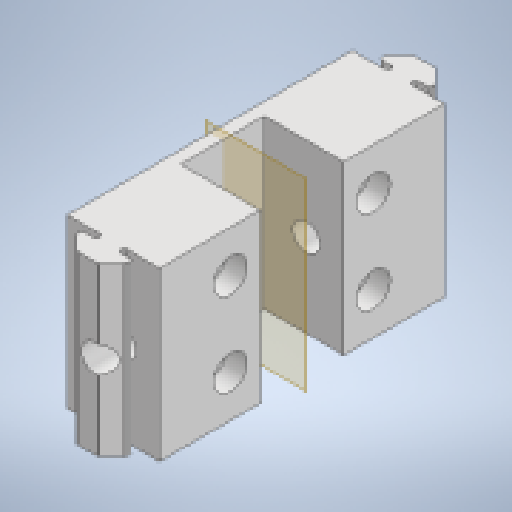
# Autodesk Inventor part: linac_upper_holder
Saved by Autodesk Inventor 2024 (Build 280153000, 153)
## iProperties
Created: 2025-12-26
Part Number: linac_upper_holder
Material: Generic
Document SubType Name: Modeling
Designer: schar
Density: 1 g/cm^3
Appearance: Default
Author: schar
Autodesk Inventor part; units mm, degrees
ref_plane "YZ Plane" through (0, 0, 0) normal (1, 0, 0) x (0, 1, 0)
ref_plane "XZ Plane" through (0, 0, 0) normal (0, 1, 0) x (-1, 0, 0)
sketch "Sketch1" plane through (0, 0, 0) normal (1, 0, 0) x (0, 1, 0)
  line L0 (20, 27.056) -> (-20, 27.056)
  line L1 (-20, 27.056) -> (-20, -27.056)
  line L2 (-20, -27.056) -> (20, -27.056)
  line L3 (20, -27.056) -> (20, 27.056)
  line L4 (20, 27.056) -> (-20, -27.056) construction
  line L5 (-20, 27.056) -> (20, -27.056) construction
  point P0 (0, 0)
  dimension "d0" = 40
  dimension "d1" = 54.112
  constraints: 12 end point, 2 midpoint, 2 parallel, 1 horizontal, 1 perpendicular
  measures "d0" distance of L2.end L1.end
  measures "d1" distance of L1.end L0.end
extrude "Extrusion1" add sketch "Sketch1" along normal blind 4
sketch "Sketch2" plane through (4, 0, 0) normal (1, 0, 0) x (0, 0, -1)
  line L0 (-9, 9) -> (9, 9)
  line L1 (9, 9) -> (9, -9)
  line L2 (9, -9) -> (-9, -9)
  line L3 (-9, -9) -> (-9, 9)
  line L4 (-9, 9) -> (9, -9) construction
  line L5 (9, 9) -> (-9, -9) construction
  line L6 (-27.056, -20) -> (27.056, -20) projected
  line L7 (-27.056, 20) -> (27.056, 20)
  line L8 (27.056, 20) -> (27.056, -20)
  line L9 (27.056, -20) -> (-27.056, -20)
  line L10 (-27.056, -20) -> (-27.056, 20)
  line L11 (-27.056, 20) -> (27.056, -20) construction
  line L12 (27.056, 20) -> (-27.056, -20) construction
  point P0 (0, 0)
  dimension "d4" = 18
  dimension "d5" = 18
  constraints: 24 end point, 4 midpoint, 4 parallel, 2 horizontal, 2 perpendicular
  measures "d4" distance of L1.end L2.end
  measures "d5" distance of L0.end L1.end
extrude "Extrusion2" add sketch "Sketch2" along normal blind 18
sketch "Sketch3" plane through (22, 0, 0) normal (1, 0, 0) x (0, 0, -1)
  line L0 (9, -9) -> (-9, -9) projected
  line L1 (-27.056, -20) -> (27.056, -20) projected
  line L2 (-9, -9) -> (9, -9)
  line L3 (9, -9) -> (9, -20)
  line L4 (9, -20) -> (-9, -20)
  line L5 (-9, -20) -> (-9, -9)
  point P0 (0, 0)
  dimension "d8" = 18
  constraints: 8 end point, 2 parallel, 1 horizontal, 1 perpendicular, 1 point on line
  measures "d8" distance of L3.end L4.end
extrude "Extrusion3" cut sketch "Sketch3" against normal blind 18
sketch "Sketch4" plane through (22, 0, 0) normal (1, 0, 0) x (0, 0, -1)
  line L0 (-27.056, 20) -> (-27.056, -20) projected
  line L1 (-27.056, -20) -> (-17.056, -20)
  line L2 (-27.056, -20) -> (27.056, -20) projected
  line L3 (-17.056, -20) -> (-17.056, -10)
  line L4 (-27.056, 20) -> (-17.056, 20)
  line L5 (27.056, 20) -> (-27.056, 20) projected
  line L6 (-17.056, 20) -> (-17.056, 10)
  line L7 (27.056, -20) -> (27.056, 20) projected
  line L8 (27.056, 20) -> (27.056, 10)
  line L9 (27.056, 10) -> (17.056, 10)
  line L10 (27.056, -20) -> (27.056, -10)
  line L11 (27.056, -10) -> (17.056, -10)
  circle A0 centre (-17.056, 10) radius 2.5
  circle A1 centre (-17.056, -10) radius 2.5
  circle A2 centre (17.056, 10) radius 2.5
  circle A3 centre (17.056, -10) radius 2.5
  point P0 (0, 0)
  dimension "d11" = 10
  dimension "d12" = 10
  dimension "d13" = 10
  dimension "d14" = 10
  dimension "d15" = 10
  dimension "d16" = 10
  dimension "d17" = 10
  dimension "d18" = 10
  dimension "d19" = 5
  dimension "d20" = 5
  dimension "d21" = 5
  dimension "d22" = 5
  constraints: 16 end point, 4 centre point, 4 coincident, 4 point on line, 3 perpendicular, 1 vertical
  measures "d11" distance of L0.end L1.end
  measures "d12" distance of L1.end L3.end
  measures "d13" distance of L0.start L4.end
  measures "d14" distance of L4.end L6.end
  measures "d15" distance of L5.start L8.end
  measures "d16" distance of L8.end L9.end
  measures "d17" distance of L2.end L10.end
  measures "d18" distance of L10.end L11.end
  measures "d19" diameter of A0
  measures "d20" diameter of A1
  measures "d21" diameter of A2
  measures "d22" diameter of A3
extrude "Extrusion4" cut sketch "Sketch4" against normal through all contours A0 | A1 | A2 | A3
sketch "Sketch6" plane through (0, -20, -27.056) normal (0, 0, -1) x (-1, 0, 0)
  line L0 (0, 20) -> (-22, 20)
  line L1 (-22, 20) -> (-13, 20)
  circle A0 centre (-13, 20) radius 3.25
  dimension "d32" = 22
  dimension "d33" = 9
  dimension "d34" = 6.5
  constraints: 4 end point, 1 centre point, 1 coincident, 1 horizontal, 1 point on line
  measures "d32" distance of L0.start L0.end
  measures "d33" distance of L0.end L1.end
  measures "d34" diameter of A0
extrude "Extrusion5" cut sketch "Sketch6" against normal through all
sketch "Sketch7" plane through (4, -20, 9) normal (0, 0, -1) x (-1, 0, 0)
  line L0 (0, 29) -> (-18, 29) projected
  line L1 (0, 0) -> (-18, 0)
  line L2 (-18, 0) -> (-18, 29)
  line L3 (-18, 29) -> (0, 29)
  line L4 (0, 29) -> (0, 0)
  point P0 (4, 20)
  constraints: 8 end point, 2 parallel, 1 horizontal, 1 perpendicular
extrude "Extrusion6" cut sketch "Sketch7" against normal blind 1
sketch "Sketch8" plane through (4, -20, -9) normal (0, 0, 1) x (1, 0, 0)
  line L0 (18, 29) -> (18, 0) projected
  line L1 (0, 29) -> (18, 29) projected
  line L2 (18, 0) -> (0, 0)
  line L3 (0, 0) -> (0, 29)
  line L4 (0, 29) -> (18, 29)
  line L5 (18, 29) -> (18, 0)
  point P0 (-4, 20)
  constraints: 8 end point, 2 parallel, 1 horizontal, 1 perpendicular
extrude "Extrusion7" cut sketch "Sketch8" against normal blind 1
sketch "Sketch9" plane through (4, 0, 0) normal (1, 0, 0) x (0, 0, -1)
  line L0 (-10, 9) -> (-10, -20) projected
  line L1 (10, -20) -> (10, 9) projected
  line L2 (-10, 9) -> (10, 9)
  line L3 (10, 9) -> (10, -20)
  line L4 (10, -20) -> (-10, -20)
  line L5 (-10, -20) -> (-10, 9)
  point P0 (0, 0)
  constraints: 8 end point, 2 parallel, 1 horizontal, 1 perpendicular
extrude "Extrusion8" cut sketch "Sketch9" against normal blind 2
sketch "Sketch10" plane through (22, 0, 0) normal (1, 0, 0) x (0, 0, -1)
  circle A0 centre (-17.056, 10) radius 2.5 projected
  circle A1 centre (-17.056, 10) radius 4
  circle A2 centre (17.056, 10) radius 2.5 projected
  circle A3 centre (17.056, 10) radius 4
  circle A4 centre (17.056, -10) radius 2.5 projected
  circle A5 centre (17.056, -10) radius 4
  circle A6 centre (-17.056, -10) radius 2.5 projected
  circle A7 centre (-17.056, -10) radius 4
  point P0 (0, 0)
  dimension "d43" = 8
  dimension "d44" = 8
  dimension "d45" = 8
  dimension "d46" = 8
  constraints: 4 centre point, 4 coincident
  measures "d43" diameter of A1
  measures "d44" diameter of A3
  measures "d45" diameter of A5
  measures "d46" diameter of A7
extrude "Extrusion9" cut sketch "Sketch10" against normal blind 5 contours A0 | A1 | A3 | A5 | A6 | A7
sketch "Sketch11" plane through (22, 9, -10) normal (0, -1, 0) x (1, 0, 0)
  line L0 (0, 0) -> (-20, 0) projected
  line L1 (0, 20) -> (-20, 20)
  line L2 (-20, 20) -> (-20, 0)
  line L3 (-20, 0) -> (0, 0)
  line L4 (0, 0) -> (0, 20)
  point P0 (-22, 10)
  constraints: 8 end point, 2 parallel, 1 horizontal, 1 perpendicular
extrude "Extrusion10" cut sketch "Sketch11" against normal through all
sketch "Sketch12" plane through (0, -20, -27.056) normal (0, 0, -1) x (-1, 0, 0)
  line L0 (0, 0) -> (0, 40) projected
  line L1 (0, 0) -> (-22, 0) projected
  line L2 (0, 40) -> (-22, 40)
  line L3 (-22, 40) -> (-22, 0)
  line L4 (-22, 0) -> (0, 0)
  line L5 (0, 0) -> (0, 40)
  circle A0 centre (-13, 20) radius 3.25 projected
  circle A1 centre (-13, 20) radius 3.25
  point P0 (0, 20)
  constraints: 8 end point, 2 parallel, 1 centre point, 1 coincident, 1 horizontal, 1 perpendicular
extrude "Extrusion11" add sketch "Sketch12" along normal blind 7
sketch "Sketch13" plane through (0, -20, 27.056) normal (0, 0, 1) x (1, 0, 0)
  circle A0 centre (13, 20) radius 3.25 projected
  circle A1 centre (13, 20) radius 3.25
  line L0 (0, 40) -> (0, 0) projected
  line L1 (0, 40) -> (22, 40) projected
  line L2 (0, 0) -> (22, 0)
  line L3 (22, 0) -> (22, 40)
  line L4 (22, 40) -> (0, 40)
  line L5 (0, 40) -> (0, 0)
  point P0 (0, 20)
  constraints: 8 end point, 2 parallel, 1 centre point, 1 coincident, 1 horizontal, 1 perpendicular
extrude "Extrusion12" add sketch "Sketch13" along normal blind 7
sketch "Sketch14" plane through (2, 20, 10) normal (0, 1, 0) x (1, 0, 0)
  arc A0 (9.804, 52.1209) -> (11.1249, 51.7515) centre (10.5684, 52.308) ccw
  line L0 (11.1249, 51.7515) -> (11.3045, 51.9311)
  arc A1 (11.3045, 51.9311) -> (10.9351, 53.252) centre (10.748, 52.4876) ccw
  arc A2 (10.9351, 53.252) -> (10.9351, 54.86) centre (9, 54.056) ccw
  arc A3 (10.9351, 54.86) -> (11.3045, 56.1809) centre (10.748, 55.6244) ccw
  line L1 (11.3045, 56.1809) -> (11.1249, 56.3605)
  arc A4 (11.1249, 56.3605) -> (9.804, 55.9911) centre (10.5684, 55.804) ccw
  arc A5 (9.804, 55.9911) -> (8.196, 55.9911) centre (9, 54.056) ccw
  arc A6 (8.196, 55.9911) -> (6.8751, 56.3605) centre (7.4316, 55.804) ccw
  line L2 (6.8751, 56.3605) -> (6.6955, 56.1809)
  arc A7 (6.6955, 56.1809) -> (7.0649, 54.86) centre (7.252, 55.6244) ccw
  arc A8 (7.0649, 54.86) -> (7.0649, 53.252) centre (9, 54.056) ccw
  arc A9 (7.0649, 53.252) -> (6.6955, 51.9311) centre (7.252, 52.4876) ccw
  line L3 (6.6955, 51.9311) -> (6.8751, 51.7515)
  arc A10 (6.8751, 51.7515) -> (8.196, 52.1209) centre (7.4316, 52.308) ccw
  arc A11 (8.196, 52.1209) -> (9.804, 52.1209) centre (9, 54.056) ccw
  line L4 (18.008, 56.686) -> (18.492, 56.686)
  arc A12 (17.5, 57.194) -> (18.008, 56.686) centre (18.008, 57.194) ccw
  line L5 (17.5, 59.543) -> (17.5, 57.194)
  arc A13 (17.5, 59.543) -> (16.992, 60.051) centre (16.992, 59.543) ccw
  line L6 (16.2661, 60.051) -> (16.992, 60.051)
  arc A14 (16.2661, 60.051) -> (15.9069, 59.9022) centre (16.2661, 59.543) ccw
  line L7 (12.8038, 56.7991) -> (15.9069, 59.9022)
  arc A15 (12.8038, 56.7991) -> (12.655, 56.4399) centre (13.163, 56.4399) ccw
  line L8 (12.655, 51.6721) -> (12.655, 56.4399)
  arc A16 (12.655, 51.6721) -> (12.8038, 51.3129) centre (13.163, 51.6721) ccw
  line L9 (15.9069, 48.2098) -> (12.8038, 51.3129)
  arc A17 (15.9069, 48.2098) -> (16.2661, 48.061) centre (16.2661, 48.569) ccw
  line L10 (16.992, 48.061) -> (16.2661, 48.061)
  arc A18 (16.992, 48.061) -> (17.5, 48.569) centre (16.992, 48.569) ccw
  line L11 (17.5, 50.918) -> (17.5, 48.569)
  arc A19 (18.008, 51.426) -> (17.5, 50.918) centre (18.008, 50.918) ccw
  line L12 (18.492, 51.426) -> (18.008, 51.426)
  arc A20 (19, 50.918) -> (18.492, 51.426) centre (18.492, 50.918) ccw
  line L13 (19, 45.556) -> (19, 50.918)
  arc A21 (17.5, 44.056) -> (19, 45.556) centre (17.5, 45.556) ccw
  line L14 (12.138, 44.056) -> (17.5, 44.056)
  arc A22 (11.63, 44.564) -> (12.138, 44.056) centre (12.138, 44.564) ccw
  line L15 (11.63, 45.048) -> (11.63, 44.564)
  arc A23 (12.138, 45.556) -> (11.63, 45.048) centre (12.138, 45.048) ccw
  line L16 (14.487, 45.556) -> (12.138, 45.556)
  arc A24 (14.487, 45.556) -> (14.995, 46.064) centre (14.487, 46.064) ccw
  line L17 (14.995, 46.7899) -> (14.995, 46.064)
  arc A25 (14.995, 46.7899) -> (14.8462, 47.1491) centre (14.487, 46.7899) ccw
  line L18 (11.7431, 50.2522) -> (14.8462, 47.1491)
  arc A26 (11.7431, 50.2522) -> (11.3839, 50.401) centre (11.3839, 49.893) ccw
  line L19 (6.6161, 50.401) -> (11.3839, 50.401)
  arc A27 (6.6161, 50.401) -> (6.2569, 50.2522) centre (6.6161, 49.893) ccw
  line L20 (3.1538, 47.1491) -> (6.2569, 50.2522)
  arc A28 (3.1538, 47.1491) -> (3.005, 46.7899) centre (3.513, 46.7899) ccw
  line L21 (3.005, 46.064) -> (3.005, 46.7899)
  arc A29 (3.005, 46.064) -> (3.513, 45.556) centre (3.513, 46.064) ccw
  line L22 (5.862, 45.556) -> (3.513, 45.556)
  arc A30 (6.37, 45.048) -> (5.862, 45.556) centre (5.862, 45.048) ccw
  line L23 (6.37, 44.564) -> (6.37, 45.048)
  arc A31 (5.862, 44.056) -> (6.37, 44.564) centre (5.862, 44.564) ccw
  line L24 (0.5, 44.056) -> (5.862, 44.056)
  arc A32 (-1, 45.556) -> (0.5, 44.056) centre (0.5, 45.556) ccw
  line L25 (-1, 50.918) -> (-1, 45.556)
  arc A33 (-0.492, 51.426) -> (-1, 50.918) centre (-0.492, 50.918) ccw
  line L26 (-0.008, 51.426) -> (-0.492, 51.426)
  arc A34 (0.5, 50.918) -> (-0.008, 51.426) centre (-0.008, 50.918) ccw
  line L27 (0.5, 48.569) -> (0.5, 50.918)
  arc A35 (0.5, 48.569) -> (1.008, 48.061) centre (1.008, 48.569) ccw
  line L28 (1.7339, 48.061) -> (1.008, 48.061)
  arc A36 (1.7339, 48.061) -> (2.0931, 48.2098) centre (1.7339, 48.569) ccw
  line L29 (5.1962, 51.3129) -> (2.0931, 48.2098)
  arc A37 (5.1962, 51.3129) -> (5.345, 51.6721) centre (4.837, 51.6721) ccw
  line L30 (5.345, 56.4399) -> (5.345, 51.6721)
  arc A38 (5.345, 56.4399) -> (5.1962, 56.7991) centre (4.837, 56.4399) ccw
  line L31 (2.0931, 59.9022) -> (5.1962, 56.7991)
  arc A39 (2.0931, 59.9022) -> (1.7339, 60.051) centre (1.7339, 59.543) ccw
  line L32 (1.008, 60.051) -> (1.7339, 60.051)
  arc A40 (1.008, 60.051) -> (0.5, 59.543) centre (1.008, 59.543) ccw
  line L33 (0.5, 57.194) -> (0.5, 59.543)
  arc A41 (-0.008, 56.686) -> (0.5, 57.194) centre (-0.008, 57.194) ccw
  line L34 (-0.492, 56.686) -> (-0.008, 56.686)
  arc A42 (-1, 57.194) -> (-0.492, 56.686) centre (-0.492, 57.194) ccw
  line L35 (-1, 62.556) -> (-1, 57.194)
  arc A43 (0.5, 64.056) -> (-1, 62.556) centre (0.5, 62.556) ccw
  line L36 (5.862, 64.056) -> (0.5, 64.056)
  arc A44 (6.37, 63.548) -> (5.862, 64.056) centre (5.862, 63.548) ccw
  line L37 (6.37, 63.064) -> (6.37, 63.548)
  arc A45 (5.862, 62.556) -> (6.37, 63.064) centre (5.862, 63.064) ccw
  line L38 (3.513, 62.556) -> (5.862, 62.556)
  arc A46 (3.513, 62.556) -> (3.005, 62.048) centre (3.513, 62.048) ccw
  line L39 (3.005, 61.3221) -> (3.005, 62.048)
  arc A47 (3.005, 61.3221) -> (3.1538, 60.9629) centre (3.513, 61.3221) ccw
  line L40 (6.2569, 57.8598) -> (3.1538, 60.9629)
  arc A48 (6.2569, 57.8598) -> (6.6161, 57.711) centre (6.6161, 58.219) ccw
  line L41 (11.3839, 57.711) -> (6.6161, 57.711)
  arc A49 (11.3839, 57.711) -> (11.7431, 57.8598) centre (11.3839, 58.219) ccw
  line L42 (14.8462, 60.9629) -> (11.7431, 57.8598)
  arc A50 (14.8462, 60.9629) -> (14.995, 61.3221) centre (14.487, 61.3221) ccw
  line L43 (14.995, 62.048) -> (14.995, 61.3221)
  arc A51 (14.995, 62.048) -> (14.487, 62.556) centre (14.487, 62.048) ccw
  line L44 (12.138, 62.556) -> (14.487, 62.556)
  arc A52 (11.63, 63.064) -> (12.138, 62.556) centre (12.138, 63.064) ccw
  line L45 (11.63, 63.548) -> (11.63, 63.064)
  arc A53 (12.138, 64.056) -> (11.63, 63.548) centre (12.138, 63.548) ccw
  line L46 (17.5, 64.056) -> (12.138, 64.056)
  arc A54 (19, 62.556) -> (17.5, 64.056) centre (17.5, 62.556) ccw
  line L47 (19, 57.194) -> (19, 62.556)
  arc A55 (18.492, 56.686) -> (19, 57.194) centre (18.492, 57.194) ccw
  line L48 (20, 44.056) -> (-2, 44.056) projected
  line L49 (9, 44.056) -> (9, 48.233)
  line L50 (5.862, 44.056) -> (12.138, 44.056)
  point P0 (-2, 10)
  point P1 (11.63, 44.564)
  point P2 (12.138, 45.556)
  point P3 (14.995, 46.064)
  point P4 (14.8462, 47.1491)
  point P5 (11.3839, 50.401)
  point P6 (6.2569, 50.2522)
  point P7 (3.005, 46.7899)
  point P8 (3.513, 45.556)
  point P9 (6.37, 44.564)
  point P10 (5.862, 44.056)
  dimension "d55" = 4.177
  constraints: 112 point on circle, 100 end point, 56 centre point, 1 collinear, 1 midpoint, 1 vertical
  measures "d55" distance of L49.start L49.end
extrude "Extrusion13" add sketch "Sketch14" against normal up to surface (40 mm away) contours L48 A31 L23 A30 L22 A29 L21 A28 L20 A27 L19 A26 L18 A25 L17 A24 L16 A23 L15 A22
ref_plane "Work Plane1" through (4, -20, 0) normal (0, 0, 1) x (1, 0, 0)
mirror "Mirror1" about plane through (4, -20, 0) normal (0, 0, 1) of "Extrusion13"
sketch "Sketch15" plane through (2, 0, 0) normal (1, 0, 0) x (0, 0, -1)
  line L0 (10, 20) -> (10, -20) projected
  line L1 (10, 20) -> (-10, 20)
  line L2 (-10, 20) -> (-10, -20)
  line L3 (-10, -20) -> (10, -20)
  line L4 (10, -20) -> (10, 20)
  point P0 (0, 0)
  constraints: 8 end point, 2 parallel, 1 horizontal, 1 perpendicular
extrude "Extrusion14" add sketch "Sketch15" along normal blind 1
sketch "Sketch16" plane through (4, -20, 10) normal (0, 0, -1) x (-1, 0, 0)
  circle A0 centre (-9, 20) radius 3.25 projected
  circle A1 centre (-9, 20) radius 3.25
  point P0 (4, 20)
  constraints: 1 centre point, 1 coincident
extrude "Extrusion15" cut sketch "Sketch16" along normal through all both and the other way through all
ref_plane "Work Plane2" through (8.6161, 20, 0) normal (0, 0, 1) x (1, 0, 0)
body "Solid1"
